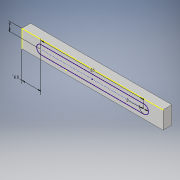
# Autodesk Inventor part: crat8
Saved by Autodesk Inventor 2019 (Build 230136000, 136)
## iProperties
Created: 2021-11-12
Part Number: crat8
Material: 一般
Document SubType Name: Sheet Metal
Designer: yuta
Density: 1 g/cm^3
Sheet Metal Rule: Default_mm
Appearance: 既定
Author: yuta
Autodesk Inventor part; units mm, degrees
ref_plane "YZ Plane" through (0, 0, 0) normal (1, 0, 0) x (0, 1, 0)
ref_plane "XZ Plane" through (0, 0, 0) normal (0, 1, 0) x (-1, 0, 0)
ref_plane "XY Plane" through (0, 0, 0) normal (0, 0, 1) x (1, 0, 0)
sketch "スケッチ1" plane through (0, 0, 0) normal (0, 0, 1) x (1, 0, 0)
  line L0 (-14.9977, 4.8641) -> (33.0023, 4.8641)
  line L1 (33.0023, 4.8641) -> (33.0023, -1.1359)
  line L2 (33.0023, -1.1359) -> (-14.9977, -1.1359)
  line L3 (-14.9977, -1.1359) -> (-14.9977, 4.8641)
  point P0 (0, 0)
  dimension "d0" = 48
  dimension "d1" = 6
  constraints: 8 end point, 2 parallel, 1 horizontal, 1 perpendicular
  measures "d0" distance of L1.end L2.end
  measures "d1" distance of L0.end L1.end
sketch "スケッチ2" plane through (0, 0, 0) normal (0, 0, 1) x (1, 0, 0)
  point P0 (0, 0)
extrude "押し出し1" add sketch "スケッチ1" along normal blind 3
sketch "スケッチ3" plane through (0, 0, 3) normal (0, 0, 1) x (1, 0, 0)
  line L0 (-8.4977, 1.8641) -> (26.5023, 1.8641) construction
  line L1 (-8.4977, 0.3641) -> (26.5023, 0.3641)
  line L2 (26.5023, 3.3641) -> (-8.4977, 3.3641)
  arc A0 (-8.4977, 3.3641) -> (-8.4977, 0.3641) centre (-8.4977, 1.8641) ccw
  arc A1 (26.5023, 0.3641) -> (26.5023, 3.3641) centre (26.5023, 1.8641) ccw
  line L3 (-14.9977, 4.8641) -> (-14.9977, -1.1359) projected
  line L4 (33.0023, 4.8641) -> (-14.9977, 4.8641) projected
  point P0 (0, 0)
  point P1 (9.0023, 1.8641)
  dimension "d4" = 35
  dimension "d5" = 3
  dimension "d6" = 6.5
  dimension "d7" = 3
  constraints: 8 end point, 4 point on circle, 4 tangent, 2 centre point, 1 horizontal, 1 midpoint, 1 parallel
  measures "d4" distance of L0.start L0.end
  measures "d5" diameter of A1
  measures "d6" distance from line of L3 L0.start
  measures "d7" distance from line of L4 L0.start
equation "\"BendRadius\" = Thickness"
equation "\"BendReliefWidth\" = Thickness"
equation "\"BendReliefDepth\" = 0.5 * Thickness"
equation "\"CornerReliefSize\" = 4 * Thickness"
equation "\"MinimumRemnant\" = 2 * Thickness"
equation "\"TransitionRadius\" = BendRadius"
equation "\"JacobiRadiusSize\" = BendRadius"
equation "\"GapSize\" = Thickness"
equation "\"Thickness\" = 0.5"
